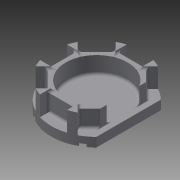
# Autodesk Inventor part: receiver mount
Saved by Autodesk Inventor 2015 (Build 190159000, 159)
## iProperties
Created: 2016-02-14
Part Number: receiver mount
Material: Generic
Document SubType Name: Modeling
Designer: -
Density: 1 g/cm^3
Appearance: Default
Author: -
Autodesk Inventor part; units mm, degrees
ref_plane "YZ Plane" through (0, 0, 0) normal (1, 0, 0) x (0, 1, 0)
ref_plane "XZ Plane" through (0, 0, 0) normal (0, 1, 0) x (-1, 0, 0)
ref_plane "XY Plane" through (0, 0, 0) normal (0, 0, 1) x (1, 0, 0)
sketch "Sketch7" plane through (0, 0, 0) normal (0, 1, 0) x (-1, 0, 0)
  circle A0 centre (0, 0) radius 26.556349
  circle A1 centre (0, 0) radius 23.556349
  circle A2 centre (0, 0) radius 34.556349
  line L0 (26.556349, 11) -> (26.556349, -11)
  line L1 (26.556349, -10.25) -> (33.001193, -10.25)
  line L2 (26.556349, 10.25) -> (33.001193, 10.25)
  line L3 (26.556349, 11) -> (11, 26.556349)
  line L4 (11, 26.556349) -> (-11, 26.556349)
  line L5 (-11, 26.556349) -> (-26.556349, 11)
  line L6 (-26.556349, 11) -> (-26.556349, -11)
  line L7 (-26.556349, -11) -> (-11, -26.556349)
  line L8 (-11, -26.556349) -> (11, -26.556349)
  line L9 (11, -26.556349) -> (26.556349, -11)
  line L10 (26.026019, 11.53033) -> (30.583212, 16.087523)
  line L11 (11.53033, 26.026019) -> (16.087523, 30.583212)
  line L12 (10.25, 26.556349) -> (10.25, 33.001193)
  line L13 (-10.25, 26.556349) -> (-10.25, 33.001193)
  line L14 (-26.026019, -11.53033) -> (-30.583212, -16.087523)
  line L15 (-11.53033, -26.026019) -> (-16.087523, -30.583212)
  line L16 (-10.25, -26.556349) -> (-10.25, -33.001193)
  line L17 (10.25, -26.556349) -> (10.25, -33.001193)
  line L18 (11.53033, -26.026019) -> (16.087523, -30.583212)
  line L19 (26.026019, -11.53033) -> (30.583212, -16.087523)
  line L20 (-26.556349, 10.25) -> (-33.001193, 10.25)
  line L21 (-26.556349, -10.25) -> (-33.001193, -10.25)
  line L22 (-26.026019, 11.53033) -> (-30.583212, 16.087523)
  line L23 (-11.53033, 26.026019) -> (-16.087523, 30.583212)
  line L24 (0, 0) -> (-13.224142, 31.925904)
  line L25 (-13.224142, -31.925904) -> (0, 0)
  line L26 (-20, 48.284271) -> (-20, -48.284271)
  point P0 (-20, 28.180512)
  point P1 (-20, -28.180512)
  point P2 (0, 26.556349)
  point P3 (18.778175, 18.778175)
  point P4 (26.556349, 0)
  point P5 (18.778175, -18.778175)
  point P6 (0, -26.556349)
  point P7 (-18.778175, -18.778175)
  point P8 (-20, -17.47111)
  point P9 (-20, -17.556349)
  point P10 (-20, -12.445947)
  point P11 (-20, 12.445947)
  point P12 (-20, 17.47111)
  point P13 (-20, 18.266998)
  point P14 (-18.778175, 18.778175)
  point P15 (-26.556349, 0)
  point P16 (-10.162675, 24.534867)
  point P17 (-9.014625, 21.763229)
  point P18 (-9.014625, -21.763229)
  point P19 (-10.162675, -24.534867)
  dimension "d67" = 8
  dimension "d66" = 3
  dimension "d69" = 135
  dimension "d70" = 22
  dimension "d71" = 0.75
  dimension "d72" = 0.75
  dimension "d73" = 0.75
  dimension "d74" = 0.75
  dimension "d75" = 0.75
  dimension "d76" = 0.75
  dimension "d77" = 0.75
  dimension "d78" = 0.75
  dimension "d79" = 0.75
  dimension "d80" = 0.75
  dimension "d81" = 0.75
  dimension "d82" = 0.75
  dimension "d83" = 0.75
  dimension "d84" = 0.75
  dimension "d85" = 0.75
  dimension "d86" = 0.75
  dimension "d87" = 20
  constraints: 52 end point, 25 point on line, 16 perpendicular, 8 midpoint, 7 equal length, 4 point on circle, 3 coincident, 3 vertical, 2 horizontal, 1 centre point, 50 other
  measures "d69" angle of L9 L0
  measures "d70" distance of L0.start L0.end
  measures "d71" distance from line of L2 L0.start
  measures "d72" distance from line of L0.end L1
  measures "d73" distance from line of L0.end L19
  measures "d74" distance from line of L17 L8.end
  measures "d75" distance from line of L7.end L16
  measures "d76" distance from line of L8.end L18
  measures "d77" distance from line of L7.end L15
  measures "d78" distance from line of L6.end L14
  measures "d79" distance from line of L6.end L21
  measures "d80" distance from line of L20 L5.end
  measures "d81" distance from line of L5.end L22
  measures "d82" distance from line of L4.end L23
  measures "d83" distance from line of L4.end L13
  measures "d84" distance from line of L3.end L12
  measures "d85" distance from line of L3.end L11
  measures "d86" distance from line of L0.start L10
sketch "Sketch8" plane through (0, 0, 0) normal (0, 1, 0) x (-1, 0, 0)
  line L0 (-20, 48.284271) -> (-20, -48.284271)
  circle A0 centre (0, 0) radius 34.556349
  line L1 (20.25, -30.25) -> (-20.25, -30.25)
  line L2 (-20.25, -30.25) -> (-20.25, 30.25)
  line L3 (-20.25, 30.25) -> (20.25, 30.25)
  line L4 (20.25, 30.25) -> (20.25, -30.25)
  line L5 (-24.25, 24.618667) -> (-24.25, -24.618667)
  line L6 (16.25, 30.25) -> (16.25, 26.25)
  line L7 (16.25, 26.25) -> (20.25, 26.25)
  line L8 (-16.25, 30.25) -> (-16.25, 26.25)
  line L9 (-16.25, 26.25) -> (-20.25, 26.25)
  line L10 (20.25, -26.25) -> (16.25, -26.25)
  line L11 (16.25, -26.25) -> (16.25, -30.25)
  line L12 (-16.25, -30.25) -> (-16.25, -26.25)
  line L13 (-20.25, -26.25) -> (-16.25, -26.25)
  point P0 (-20.25, 28.001407)
  point P1 (-20.25, -28.001407)
  point P2 (-16.705651, -30.25)
  point P3 (16.705651, -30.25)
  point P4 (20.25, -28.001407)
  point P5 (20.25, 28.001407)
  point P6 (16.705651, 30.25)
  point P7 (-16.705651, 30.25)
  point P8 (-20, 28.180512)
  point P9 (-20, -28.180512)
  dimension "d114" = 20.25
  dimension "d115" = 20.25
  dimension "d116" = 30.25
  dimension "d117" = 30.25
  dimension "d118" = 4
  dimension "d123" = 4
  dimension "d124" = 4
  dimension "d125" = 4
  dimension "d126" = 4
  constraints: 26 end point, 26 point on line, 4 perpendicular, 3 parallel, 2 vertical, 1 horizontal, 13 other
  measures "d114" distance from line of L4 point (0, 0)
  measures "d115" distance from line of L2 point (0, 0)
  measures "d116" distance from line of L1 point (0, 0)
  measures "d117" distance from line of L3 point (0, 0)
  measures "d118" distance between parallel lines of L2 L5
  measures "d123" distance of L6.end L7.end
  measures "d124" distance of L6.start L6.end
  measures "d125" distance of L13.start L12.end
  measures "d126" distance of L12.start L12.end
sketch "Sketch9" plane through (0, 0, 0) normal (0, 1, 0) x (-1, 0, 0)
  circle A0 centre (0, 0) radius 34.556349
  line L0 (-11.53033, 26.026019) -> (-16.087523, 30.583212)
  line L1 (-10.25, 26.556349) -> (-10.25, 33.001193)
  line L2 (10.25, 26.556349) -> (10.25, 33.001193)
  line L3 (11.53033, 26.026019) -> (16.087523, 30.583212)
  line L4 (26.026019, 11.53033) -> (30.583212, 16.087523)
  line L5 (26.556349, 10.25) -> (33.001193, 10.25)
  line L6 (26.556349, -10.25) -> (33.001193, -10.25)
  line L7 (26.026019, -11.53033) -> (30.583212, -16.087523)
  line L8 (11.53033, -26.026019) -> (16.087523, -30.583212)
  line L9 (10.25, -26.556349) -> (10.25, -33.001193)
  line L10 (-10.25, -26.556349) -> (-10.25, -33.001193)
  line L11 (-26.026019, -11.53033) -> (-30.583212, -16.087523)
  line L12 (-26.556349, -10.25) -> (-33.001193, -10.25)
  line L13 (-26.556349, 10.25) -> (-33.001193, 10.25)
  line L14 (-26.026019, 11.53033) -> (-30.583212, 16.087523)
  line L15 (-11.53033, -26.026019) -> (-16.087523, -30.583212)
  line L16 (11.53033, 26.026019) -> (10.25, 24.745689)
  line L17 (10.25, 24.745689) -> (10.25, 26.556349)
  line L18 (-11.53033, 26.026019) -> (-10.25, 24.745689)
  line L19 (-10.25, 24.745689) -> (-10.25, 26.556349)
  line L20 (-26.026019, 11.53033) -> (-24.745689, 10.25)
  line L21 (-24.745689, 10.25) -> (-26.556349, 10.25)
  line L22 (-26.556349, -10.25) -> (-24.745689, -10.25)
  line L23 (-24.745689, -10.25) -> (-26.026019, -11.53033)
  line L24 (-10.25, -24.745689) -> (-10.25, -26.556349)
  line L25 (10.25, -26.556349) -> (10.25, -24.745689)
  line L26 (10.25, -24.745689) -> (11.53033, -26.026019)
  line L27 (26.026019, -11.53033) -> (24.745689, -10.25)
  line L28 (24.745689, -10.25) -> (26.556349, -10.25)
  line L29 (26.556349, 10.25) -> (24.745689, 10.25)
  line L30 (26.026019, 11.53033) -> (24.745689, 10.25)
  line L31 (-10.25, -24.745689) -> (-11.53033, -26.026019)
  constraints: 32 end point, 16 collinear, 1 other
extrude "Extrusion9" add sketch "Sketch7" along normal blind 3 contours A0 L25 A1 L24 | L0 L9 A0 | A0 L3 L0 | L0 L2 A2 L1 | L3 L11 A2 L10 | A0 L4 L3 | L9 L8 A0 | L9 L19 A2 L18 | L0 L3 L10 A2 L2 | L1 A2 L19 L9 L0 | L4 L13 A2 L12 | A0 L24 L4 | L3 L4 L12 A2 L11 | L8 L25 A0 | L8 L17 A2 L16 | L18 A2 L17 L8 L9 | L24 A1 L26 A0 | A0 L5 L24 | L4 L24 A2 L13 | L25 L7 A0 | A0 L26 A1 L25 | L16 A2 L25 L8 | L5 L26 A2 L23 | A0 L26 L5 | L24 L25 A1 L26 | A1 L25 L24 | L5 L23 A2 L24 | L7 L15 A2 L26 | L25 A2 L15 L7
extrude "Extrusion10" add sketch "Sketch7" along normal blind 16 contours A0 L25 A1 L24 | L0 L9 A0 | A0 L3 L0 | A0 L4 L3 | L9 L8 A0 | L0 L3 L10 A2 L2 | L1 A2 L19 L9 L0 | A0 L24 L4 | L3 L4 L12 A2 L11 | L8 L25 A0 | L18 A2 L17 L8 L9 | L24 A1 L26 A0 | A0 L5 L24 | L4 L24 A2 L13 | L25 L7 A0 | A0 L26 A1 L25 | L16 A2 L25 L8 | L5 L23 A2 L24 | L7 L26 A0 | L25 A2 L15 L7
extrude "Extrusion11" add sketch "Sketch9" along normal blind 18 contours L5 L29 L30 L4 A0 | A0 L7 L27 L28 L6 | L3 L16 L17 L2 A0 | A0 L9 L25 L26 L8 | L1 L19 L18 L0 A0 | A0 L15 L31 L24 L10
fillet "Fillet4" radius 2 19 edges at (15.7652, 3, -21.7912) (11.5303, 9.5, -26.026) (19.4001, 3, 18.1349) (15.1543, 3, 22.4021) (11.5303, 9.5, 26.026) (10.25, 9.5, 26.5563) (0, 3, 26.5563) (-18.7782, 3, 18.7782) (-26.026, 9.5, 11.5303) (-10.25, 9.5, 26.5563) (-26.5563, 9.5, -10.25) (-26.5563, 3, 0) (-26.5563, 9.5, 10.25) (-18.7782, 3, -18.7782) (-26.026, 9.5, -11.5303) (-11.5303, 9.5, -26.026) (-10.25, 9.5, -26.5563) (0, 3, -26.5563) (10.25, 9.5, -26.5563)
fillet "Fillet5" radius 2 1 edges at (-23.5563, 3, 0)
fillet "Fillet6" radius 2 12 edges at (10.25, 16, 26.651) (-10.8902, 16, 25.3859) (-26.651, 16, 10.25) (-11.5973, 16, -26.093) (10.25, 16, -26.651) (11.5973, 16, 26.093) (11.5973, 16, -26.093) (-10.25, 16, -26.651) (-10.25, 16, 26.651) (-26.093, 16, 11.5973) (-26.093, 16, -11.5973) (-26.651, 16, -10.25)
extrude "Extrusion13" add sketch "Sketch8" along normal blind 3 contours L0 L9 L2 A0 | L0 L13 L2 L9 | L2 A0 L5 | L0 A0 L2 L13
extrude "Extrusion14" add sketch "Sketch8" against normal blind 4 contours A0 L3 | L2 A0 L5 | A0 L4 | L1 A0
extrude "Extrusion15" add sketch "Sketch8" against normal blind 2 contours A0 L3 L8 L9 L0 | L0 L9 L2 A0 | A0 L4 L7 L6 L3 | L13 L12 L1 A0 L0 | L0 A0 L2 L13 | A0 L1 L11 L10 L4
chamfer "Chamfer6" distance 1.5 angle 45 12 edges at (-20.25, 0, 0) (-18.25, 0, 26.25) (-16.25, 0, 28.25) (0, 0, 30.25) (-16.25, 0, -28.25) (16.25, 0, 28.25) (20.25, 0, 0) (18.25, 0, -26.25) (16.25, 0, -28.25) (0, 0, -30.25) (-18.25, 0, -26.25) (18.25, 0, 26.25)
body "Solid5"
